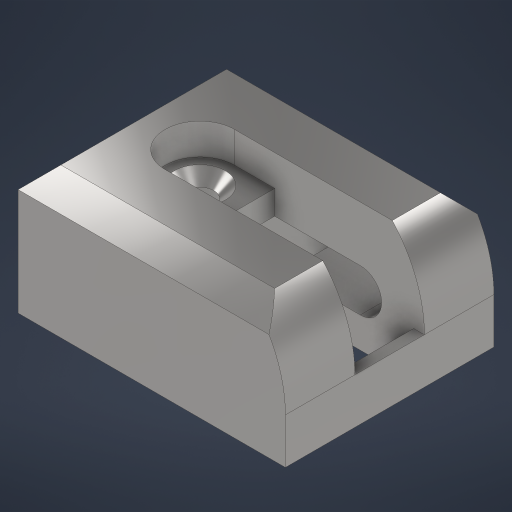
# Autodesk Inventor part: Part2
Saved by Autodesk Inventor 2023 (Build 270158000, 158)
## iProperties
Created: 2022-11-28
Part Number: Part2
Material: Steel, Carbon
Document SubType Name: Modeling
Designer: iusti
Density: 7.85 g/cm^3
Appearance: Semi-Polished
Author: iusti
Autodesk Inventor part; units mm, degrees
ref_plane "YZ Plane" through (0, 0, 0) normal (1, 0, 0) x (0, 1, 0)
ref_plane "XZ Plane" through (0, 0, 0) normal (0, 1, 0) x (-1, 0, 0)
ref_plane "XY Plane" through (0, 0, 0) normal (0, 0, 1) x (1, 0, 0)
sketch "Sketch1" plane through (0, 0, 0) normal (0, 0, 1) x (1, 0, 0)
  line L0 (0, 0) -> (50, 0)
  line L1 (50, 0) -> (50, 8.5)
  arc A0 (50, 8.5) -> (43.9926, 24) centre (27, 8.5) ccw
  line L2 (43.9926, 24) -> (0, 24)
  line L3 (0, 24) -> (0, 0)
  dimension "d3" = 50
  dimension "d4" = 24
  dimension "d5" = 23
  dimension "d6" = 8.5
  constraints: 8 end point, 3 perpendicular, 2 point on circle, 1 centre point, 1 horizontal, 1 tangent
  measures "d3" distance of L0.start L0.end
  measures "d4" distance of L2.end L0.start
  measures "d5" radius of A0
  measures "d6" distance from line of L0 A0.centre
extrude "Extrusion1" add sketch "Sketch1" along normal mid plane 39
sketch "Sketch2" plane through (0, 0, 0) normal (0, 0, 1) x (1, 0, 0)
  line L0 (0, 0) -> (0, 24) projected
  line L1 (0, 13.7) -> (38, 13.7)
  arc A0 (38, 5.7) -> (38, 13.7) centre (38, 9.7) ccw
  line L2 (38, 5.7) -> (24, 5.7)
  line L3 (24, 5.7) -> (24, 0)
  line L4 (50, 0) -> (0, 0) projected
  line L5 (24, 0) -> (0, 0)
  line L6 (0, 0) -> (0, 13.7)
  dimension "d9" = 5.7
  dimension "d10" = 26
  dimension "d11" = 4
  dimension "d12" = 38
  constraints: 10 end point, 3 perpendicular, 2 point on circle, 2 tangent, 1 centre point, 1 horizontal, 1 parallel, 1 point on line
  measures "d9" distance of L2.end L3.end
  measures "d10" distance from line of L4.start L3
  measures "d11" radius of A0
  measures "d12" distance from line of A0.centre L0
extrude "Extrusion2" cut sketch "Sketch2" along normal mid plane 31
sketch "Sketch3" plane through (0, 0, 0) normal (0, 0, 1) x (1, 0, 0)
  line L0 (0, 24) -> (43.9926, 24) projected
  line L1 (8, 24) -> (8, 18.2)
  line L2 (8, 18.2) -> (22, 18.2)
  line L3 (22, 18.2) -> (22, 0)
  line L4 (50, 0) -> (0, 0) projected
  line L5 (45, 0) -> (48, 8.5)
  line L6 (48, 8.5) -> (50, 8.5)
  line L7 (50, 8.5) -> (50, 0) projected
  line L8 (50, 24) -> (50, 8.5)
  line L9 (8, 24) -> (50, 24)
  line L10 (0, 13.7) -> (38, 13.7) projected
  dimension "d15" = 4.5
  dimension "d16" = 5
  dimension "d17" = 2
  dimension "d19" = 8.5
  dimension "d20" = 42
  dimension "d31" = 28
  constraints: 14 end point, 5 point on line, 4 perpendicular, 1 collinear
  measures "d15" distance between parallel lines of L2 L10
  measures "d16" distance of L4.start L5.start
  measures "d17" distance of L5.end L6.end
  measures "d19" distance of L4.start L6.end
  measures "d20" distance between parallel lines of L1 L8
  measures "d31" distance between parallel lines of L7 L3
extrude "Extrusion3" cut sketch "Sketch3" along normal mid plane 13 contours L0 L9 L8 L6 L5 L4 L3 L2 L1
fillet "Fillet1" radius 6.5 2 edges at (8, 21.1, 6.5) (8, 21.1, -6.5)
sketch "Sketch4" plane through (22, 18.2, 6.5) normal (0, 1, 0) x (1, 0, 0)
  arc A0 (-7.5, 13) -> (-7.5, 0) centre (-7.5, 6.5) ccw projected
  point P0 (-22, 6.5)
  constraints: 1 coincident
hole "Hole1" at (14.5, 18.2, 0) direction (0, -1, 0) diameter 5.2 end through all countersink diameter 9.5 countersink angle 90
chamfer "Chamfer1" distance 4 angle 45 3 edges at (0, 24, 0) (21.9963, 24, -19.5) (21.9963, 24, 19.5)
body "Solid1"
